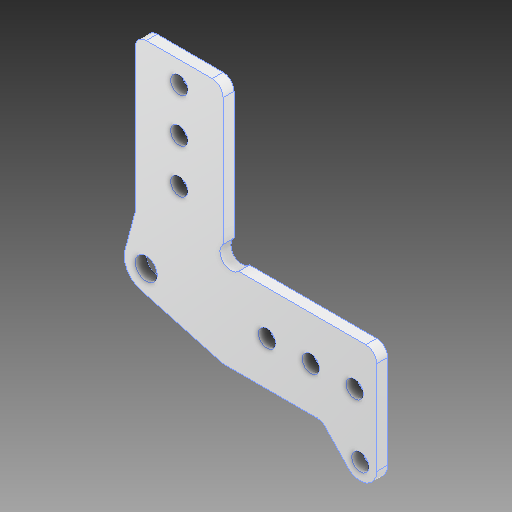
# Autodesk Inventor part: Bottom Bearing Plate Final (R4A - 0.25in Between Stages)
Saved by Autodesk Inventor 2022 (Build 260153000, 153)
## iProperties
Created: 2020-09-04
Part Number: Bottom Bearing Plate Final (R4A - 0.25in Between Stages)
Material: Aluminum 6061
Document SubType Name: Modeling
Density: 2.7 g/cm^3
Appearance: Aluminum - Flat
Autodesk Inventor part; units mm, degrees
ref_plane "YZ Plane" through (0, 0, 0) normal (1, 0, 0) x (0, 1, 0)
ref_plane "XZ Plane" through (0, 0, 0) normal (0, 1, 0) x (-1, 0, 0)
ref_plane "XY Plane" through (0, 0, 0) normal (0, 0, 1) x (1, 0, 0)
sketch "Sketch1" plane through (0, 0, 0) normal (0, 0, 1) x (1, 0, 0)
  line L0 (0, 0) -> (0, 13.4062) construction
  line L1 (0, 0) -> (20.3742, 0) construction
  circle A0 centre (9.525, 12.7) radius 9.525 construction
  circle A1 centre (9.525, 12.7) radius 3.2004
  arc A2 (3.3908, 14.3415) -> (7.8407, 6.5775) centre (9.525, 12.7) ccw
  line L2 (31.75, 0) -> (76.2, 0)
  line L3 (76.2, 0) -> (76.2, 25.4)
  line L4 (76.2, 25.4) -> (31.75, 25.4)
  line L5 (31.75, 25.4) -> (31.75, 31.75)
  line L6 (31.75, 31.75) -> (31.75, 31.75)
  line L7 (31.75, 31.75) -> (31.75, 69.85)
  line L8 (31.75, 69.85) -> (6.35, 69.85)
  line L9 (6.35, 69.85) -> (6.35, 25.4)
  line L10 (6.35, 25.4) -> (3.3908, 14.3415)
  circle A3 centre (19.05, 63.5) radius 2.4892
  circle A4 centre (19.05, 50.8) radius 2.4892
  circle A5 centre (19.05, 38.1) radius 2.4892
  circle A6 centre (44.45, 12.7) radius 2.4892
  circle A7 centre (57.15, 12.7) radius 2.4892
  circle A8 centre (69.85, 12.7) radius 2.4892
  line L11 (31.75, 31.75) -> (31.75, 25.4)
  line L12 (31.75, 25.4) -> (31.75, 25.4)
  line L13 (31.75, 0) -> (7.8407, 6.5775)
  arc A9 (67.9888, -8.047) -> (76.2, -4.7625) centre (71.4375, -4.7625) ccw
  circle A10 centre (71.4375, -4.7625) radius 2.4892
  line L14 (76.2, -4.7625) -> (76.2, 0)
  line L15 (67.9888, -8.047) -> (60.325, 0)
  arc A11 (31.75, 29.8901) -> (36.2401, 25.4) centre (33.9951, 27.6451) ccw
  circle A12 centre (31.2871, 27.4957) radius 0.4629 construction
  circle A13 centre (33.8457, 24.9371) radius 0.4629 construction
  line L16 (31.2871, 27.4957) -> (31.75, 25.4) construction
  line L17 (31.75, 25.4) -> (33.8457, 24.9371) construction
  point P0 (76.2, 12.7)
  point P1 (19.05, 69.85)
  dimension "d0" = 19.05
  dimension "d2" = 6.4008
  dimension "d6" = 12.7
  dimension "d7" = 25.4
  dimension "d8" = 4.9784
  dimension "d11" = 12.7
  dimension "d16" = 6.35
  dimension "d17" = 25.4
  dimension "d19" = 6.35
  dimension "d20" = 12.7
  dimension "d21" = 6.35
  dimension "d24" = 12.7
  dimension "d29" = 6.35
  dimension "d30" = 12.7
  dimension "d35" = 25.4
  dimension "d36" = 9.525
  dimension "d37" = 4.9784
  dimension "d38" = 3.175
  dimension "d39" = 15.875
  dimension "d40" = 6.35
  constraints: 36 end point, 14 centre point, 10 tangent, 8 perpendicular, 7 point on circle, 4 vertical, 3 coincident, 3 horizontal, 3 point on line, 2 equal radius, 2 horizontal alignment, 2 midpoint, 2 vertical alignment, 1 collinear, 1 equal length, 8 other
  measures "d0" diameter of A0
  measures "d2" diameter of A1
  measures "d6" diameter of A2
  measures "d7" distance between parallel lines of L9 L5
  measures "d8" diameter of A3
  measures "d11" distance of A3.centre A4.centre
  measures "d16" distance from line of L8 A3.centre
  measures "d17" distance between parallel lines of L2 L4
  measures "d19" distance between parallel lines of L0 L9
  measures "d20" distance from line of L4 A5.centre
  measures "d21" distance between parallel lines of L4 L6
  measures "d24" distance of A6.centre A7.centre
  measures "d29" distance from line of A8.centre L3
  measures "d30" horizontal distance of L4.end A6.centre
  measures "d35" distance between parallel lines of L9 L7
  measures "d36" diameter of A9
  measures "d37" diameter of A10
  measures "d38" distance edge to line of A0 L1
  measures "d39" distance of L2.end L15.end
  measures "d40" diameter of A11
extrude "Extrusion1" add sketch "Sketch1" along normal blind 3.175 contours L10 L9 L8 L7 L5 A11 L4 L3 L2 L13 A2 | L2 L14 A9 L15
fillet "Fillet1" radius 3.175 6 edges at (6.35, 69.85, 1.5875) (31.75, 69.85, 1.5875) (76.2, 25.4, 1.5875) (6.35, 25.4, 1.5875) (31.75, 0, 1.5875) (60.325, 0, 1.5875)
equation "\"d24\" = d11"
body "Solid1"
